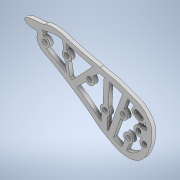
# Autodesk Inventor part: Component26
Saved by Autodesk Inventor 2022 (Build 260153000, 153)
## iProperties
Created: 2022-01-29
Part Number: Component26
Material: Generic
Document SubType Name: Modeling
Designer: Administrator
Density: 1 g/cm^3
Appearance: Default
Title: Component26
Author: Administrator
Autodesk Inventor part; units mm, degrees
ref_plane "YZ Plane" through (0, 0, 0) normal (1, 0, 0) x (0, 1, 0)
ref_plane "XZ Plane" through (0, 0, 0) normal (0, 1, 0) x (-1, 0, 0)
ref_plane "XY Plane" through (0, 0, 0) normal (0, 0, 1) x (1, 0, 0)
sketch "Sketch4" plane through (0, 0, 0) normal (0, 0, 1) x (1, 0, 0)
  circle A0 centre (-123.2659, 62.3625) radius 3.25
  circle A1 centre (-93.6225, 61.5254) radius 3.25
  circle A2 centre (-63.1067, 48.9642) radius 3.25
  circle A3 centre (-41.8815, 23.3302) radius 6.6019
  circle A4 centre (-41.8815, 23.3302) radius 3.25
  circle A5 centre (-63.1067, 48.9642) radius 6.8839
  circle A6 centre (-93.6225, 61.5254) radius 6.35
  circle A7 centre (-123.2659, 62.3625) radius 6.35
  circle A8 centre (-17.9295, 30.4928) radius 3.25
  circle A9 centre (-17.9295, 30.4928) radius 6.3607
  arc A10 (-9.0364, 0.4347) -> (-15.1641, 2.1132) centre (-10.6476, 6.5768) ccw
  circle A11 centre (-10.6476, 6.5768) radius 3.25
  circle A12 centre (-10.6476, 6.5768) radius 6.35
  circle A13 centre (3.2167, 21.804) radius 3.25
  circle A14 centre (3.2167, 21.804) radius 6.3938
  circle A15 centre (11.1828, 10.2103) radius 3.25
  circle A16 centre (11.1828, 10.2103) radius 6.35
  line L0 (0.487, 42.0553) -> (6.4199, 38.5891) construction
  line L1 (0.487, 42.0553) -> (6.4199, 38.5891) construction
  line L2 (-99.3839, 77.1398) -> (-97.7962, 66.3111)
  line L3 (-99.3839, 77.1398) -> (-97.7962, 66.3111)
  line L4 (-94.4581, 75.1449) -> (-93.4037, 67.8716)
  line L5 (-94.4581, 75.1449) -> (-93.4037, 67.8716)
  line L6 (-89.1475, 38.513) -> (-91.9311, 53.8666)
  line L7 (-92.1978, 55.3373) -> (-89.1475, 38.513)
  line L8 (-44.7292, 29.2864) -> (-43.2829, 61.21)
  line L9 (-43.2829, 61.21) -> (-44.7292, 29.2864)
  line L10 (-37.6136, 1.1054) -> (-18.29, 54.3043)
  line L11 (-16.6773, 36.7291) -> (-11.0974, 52.1068)
  line L12 (-11.0974, 52.1068) -> (-16.6773, 36.7291)
  line L13 (-30.4763, -2.5717) -> (-20.5684, 24.7053)
  line L14 (-20.5684, 24.7053) -> (-30.4763, -2.5717)
  line L15 (-15.1641, 2.1132) -> (-18.9648, -7.672)
  line L16 (-15.1641, 2.1132) -> (-18.9648, -7.672)
  line L17 (-12.6206, -8.9306) -> (-9.0364, 0.4347)
  line L18 (-9.0364, 0.4347) -> (-12.6206, -8.9306)
  spline S0 degree 1 poles (-89.1475, 38.513) (-86.314, 36.5681) knots 0 0 1 1
  spline S1 degree 3 poles (-94.4581, 75.1449) (-89.0039, 73.5308) (-61.0651, 66.1302) (-58.348, 66.0513) knots 0 0 0 0 1 1 1 1
  spline S2 degree 2 poles (-124.9306, 68.4904) (-124.7941, 71.5671) (-126.6326, 74.9703) knots 0 0 0 1 1 1
  spline S3 degree 4 poles (-126.6326, 74.9703) (-124.6811, 75.0735) (-123.6465, 74.6991) (-116.9052, 77.5165) (-111.8408, 77.8952) (-106.9644, 78.3944) (-102.5411, 77.5396) (-100.8183, 77.334) (-99.3839, 77.1398) knots 0 0 0 0 0 0.325065 0.476889 0.636712 0.785428 1 1 1 1 1
  line L19 (-102.3701, 77.544) -> (-96.3977, 76.7356) construction
  arc A17 (-96.9973, 76.8008) -> (-101.7747, 77.4475) centre (-124.0221, -104.8878) ccw construction
  spline S4 degree 4 poles (-79.9023, 31.8379) (-68.677, 24.1558) (-65.7048, 21.8411) (-54.4696, 13.1783) (-47.2097, 8.1156) knots 0 0 0 0 0 1 1 1 1 1
  line L20 (-36.0787, 59.4886) -> (-37.5047, 28.2728)
  spline S5 degree 1 poles (-50.2018, 62.6533) (-43.2829, 61.21) knots 0 0 1 1
  line L21 (-58.8336, 54.3613) -> (-50.2018, 62.6533)
  spline S6 degree 4 poles (-48.4944, 70.2012) (-36.0141, 65.7072) (-30.7305, 68.7389) (-7.2655, 57.0667) (9.3089, 53.4776) (21.1008, 36.626) (20.9729, 33.2176) (20.9498, 16.3118) (19.6092, 12.859) (15.3586, 0.2622) (11.6074, -5.1677) (4.6087, -13.37) (-6.6845, -16.5209) (-13.4963, -16.6569) (-26.6726, -14.6721) (-37.9818, -6.8681) (-48.5195, -2.2945) (-56.5284, 5.7043) (-68.3866, 14.707) (-76.2345, 20.2103) (-90.2288, 29.4992) (-101.4213, 37.2305) (-118.0489, 46.4365) (-128.5275, 50.5525) (-133.6617, 58.8987) (-134.3025, 63.1982) (-132.382, 69.7186) (-133.4886, 70.4797) (-138.3156, 70.5557) (-142.305, 70.8214) (-145.7075, 71.2674) (-149.1406, 73.4071) (-150.5992, 74.9837) (-150.3106, 77.5083) (-148.4094, 78.2404) (-147.041, 79.3341) (-144.1806, 80.1808) (-141.6683, 80.7774) (-137.5469, 81.2031) (-134.4054, 81.6387) (-131.7323, 81.4914) (-129.0357, 81.5666) (-125.9455, 82.1526) (-124.1195, 82.6025) (-123.0686, 83.1991) knots 0 0 0 0 0 0.084441 0.118474 0.150262 0.180443 0.207707 0.233569 0.259946 0.285424 0.312388 0.338232 0.365444 0.393991 0.422871 0.453116 0.483798 0.513365 0.543967 0.576006 0.609621 0.643558 0.675095 0.702806 0.725607 0.743321 0.759311 0.775075 0.790518 0.807822 0.823963 0.838322 0.851216 0.862814 0.874845 0.887711 0.90222 0.917813 0.933276 0.94829 0.962767 0.97721 1 1 1 1 1
  line L22 (-67.7671, 43.8978) -> (-79.9023, 31.8379)
  line L23 (-96.2693, 55.7533) -> (-93.9578, 41.2636)
  spline S7 degree 4 poles (-121.1299, 56.3826) (-112.9596, 50.6322) (-106.8288, 48.999) (-98.1791, 43.4387) (-93.9578, 41.2636) knots 0 0 0 0 0 1 1 1 1 1
  spline S8 degree 3 poles (-36.0787, 59.4886) (-32.0611, 58.7648) (-23.4035, 55.5205) (-18.29, 54.3043) knots 0 0 0 0 1 1 1 1
  line L24 (-38.7053, 2.6027) -> (-38.0024, 17.9881)
  spline S9 degree 4 poles (-123.0686, 83.1991) (-121.5996, 84.0331) (-117.1799, 84.5502) (-116.7574, 85.3349) (-102.0621, 84.8359) (-94.4012, 81.5385) (-82.7685, 78.513) (-69.5272, 74.408) (-54.1219, 71.5671) (-48.4944, 70.2012) knots 0 0 0 0 0 0.116866 0.21775 0.322652 0.463158 0.611266 1 1 1 1 1
  line L25 (-122.3958, 83.8471) -> (-111.8454, 85.6152) construction
  arc A18 (-112.8875, 85.1999) -> (-121.2753, 83.7942) centre (-110.8052, 47.0461) ccw construction
  line L26 (13.5332, 27.0791) -> (5.6, 27.7371)
  spline S10 degree 3 poles (13.5332, 27.0791) (17.0401, 28.2955) (11.4801, 33.321) (12.1713, 35.8976) knots 0 0 0 0 1 1 1 1
  spline S11 degree 4 poles (-12.6206, -8.9306) (-11.0988, -9.1567) (-7.9065, -8.9799) (-0.7866, -6.5594) (4.7218, -1.6082) (7.094, 3.0589) (8.3854, 4.5096) knots 0 0 0 0 0 0.301338 0.510276 1 1 1 1 1
  line L27 (-47.2097, 8.1156) -> (-46.7199, 18.8384)
  spline S12 degree 1 poles (-38.7053, 2.6027) (-37.6136, 1.1054) knots 0 0 1 1
  spline S13 degree 4 poles (-30.4763, -2.5717) (-29.8635, -4.0953) (-23.7582, -5.4905) (-22.3176, -7.1502) (-18.9648, -7.672) knots 0 0 0 0 0 1 1 1 1 1
  line L28 (0.487, 42.0553) -> (6.4199, 38.5891) construction
  line L29 (-2.7162, 36.5725) -> (3.2167, 33.1063)
  line L30 (9.6232, 44.072) -> (3.6902, 47.5382)
  arc A19 (3.6902, 47.5382) -> (-2.7162, 36.5725) centre (0.487, 42.0553) ccw
  arc A20 (3.2167, 33.1063) -> (9.6232, 44.072) centre (6.4199, 38.5891) ccw
  spline S14 degree 4 poles (-11.0974, 52.1068) (-10.8972, 52.6451) (-5.9101, 48.9599) (-3.1879, 49.4055) (-2.1589, 47.8278) knots 0 0 0 0 0 1 1 1 1 1
  line L31 (0.487, 42.0553) -> (6.4199, 38.5891) construction
  line L32 (2.1265, 44.8615) -> (8.0594, 41.3953)
  line L33 (4.7805, 35.7829) -> (-1.1524, 39.2491)
  arc A21 (2.1265, 44.8615) -> (-1.1524, 39.2491) centre (0.487, 42.0553) ccw
  arc A22 (4.7805, 35.7829) -> (8.0594, 41.3953) centre (6.4199, 38.5891) ccw
  line L34 (-86.314, 36.5681) -> (-58.348, 66.0513)
  line L35 (3.2167, 15.4102) -> (7.5381, 15.4102)
  line L36 (-15.1406, -8.5562) -> (-10.1007, -9.3049) construction
  arc A23 (-14.5441, -8.404) -> (-10.6272, -8.9859) centre (-11.3942, -0.6747) ccw construction
  point P0 (0, 0)
  point P1 (3.4535, 40.3222)
  point P2 (3.4535, 40.3222)
  point P3 (-83.197, 72.0665)
  point P4 (-63.3289, 67.0346)
  point P5 (-125.2394, 71.4578)
  point P6 (-124.5026, 75.0553)
  point P7 (-121.6588, 75.6416)
  point P8 (-116.0905, 77.2602)
  point P9 (-111.6668, 77.9259)
  point P10 (-107.1522, 78.0845)
  point P11 (-102.5828, 77.5823)
  point P12 (-63.3283, 19.9895)
  point P13 (-67.6095, 14.019)
  point P14 (-70.2118, 25.0604)
  point P15 (-55.2549, 13.9519)
  point P16 (-33.4871, 66.5925)
  point P17 (-20.6666, 63.2711)
  point P18 (-3.0393, 56.784)
  point P19 (10.3795, 49.6099)
  point P20 (19.697, 37.3317)
  point P21 (20.9543, 30.7069)
  point P22 (20.585, 17.8397)
  point P23 (19.1683, 11.5104)
  point P24 (15.3531, 1.4868)
  point P25 (11.1804, -5.3901)
  point P26 (3.8615, -12.2784)
  point P27 (-5.9583, -15.9225)
  point P28 (-13.5398, -16.304)
  point P29 (-25.3402, -13.8592)
  point P30 (-38.1309, -7.3256)
  point P31 (-48.0759, -1.557)
  point P32 (-57.007, 5.6696)
  point P33 (-76.3522, 20.2082)
  point P34 (-88.7766, 28.5824)
  point P35 (-102.5781, 37.5478)
  point P36 (-119.6247, 46.8159)
  point P37 (-129.4025, 53.2681)
  point P38 (-133.3877, 59.7383)
  point P39 (-133.6123, 64.9346)
  point P40 (-132.9983, 69.4096)
  point P41 (-133.7787, 70.2207)
  point P42 (-137.5911, 70.5697)
  point P43 (-142.3147, 70.8802)
  point P44 (-146.1131, 71.7837)
  point P45 (-149.2626, 73.7357)
  point P46 (-150.3083, 75.4489)
  point P47 (-149.9428, 77.2311)
  point P48 (-148.6086, 78.2495)
  point P49 (-147.089, 79.1182)
  point P50 (-144.6312, 80.0215)
  point P51 (-141.6917, 80.6837)
  point P52 (-137.4889, 81.2333)
  point P53 (-134.1664, 81.5354)
  point P54 (-131.7413, 81.5337)
  point P55 (-129.4102, 81.6346)
  point P56 (-126.1766, 82.1503)
  point P57 (-98.1366, 43.5746)
  point P58 (-104.7791, 47.205)
  point P59 (-112.3268, 51.1181)
  point P60 (-24.4257, 56.0733)
  point P61 (-31.6333, 58.3402)
  point P62 (-61.0372, 72.9432)
  point P63 (-86.731, 79.4913)
  point P64 (-106.3338, 84.6959)
  point P65 (-117.1206, 84.7312)
  point P66 (-94.4887, 81.835)
  point P67 (-76.4524, 76.6451)
  point P68 (14.6933, 28.7644)
  point P69 (13.081, 32.5705)
  point P70 (-25.3388, -5.3867)
  point P71 (-21.946, -6.8042)
  point P72 (6.3564, 1.6685)
  point P73 (2.6486, -2.8719)
  point P74 (-2.5579, -6.6485)
  point P75 (-12.666, -8.9237)
  point P76 (-29.0617, -3.7189)
  point P77 (3.4535, 40.3222)
  point P78 (-10.7812, 52.1086)
  point P79 (-7.5998, 50.59)
  point P80 (-3.665, 48.9029)
  point P81 (3.4535, 40.3222)
  point P82 (-44.45, 61.9125)
  point P83 (-92.0343, 55.4942)
  point P84 (12.1713, 35.8976)
  point P85 (8.2264, 4.5905)
  point P86 (-12.666, -8.7985)
  point P87 (-18.9648, -7.672)
  point P88 (-31.4568, -2.4563)
  point P89 (-120.9781, 56.439)
  point P90 (-18.8701, 54.5151)
  point P91 (-38.1296, 1.4925)
  dimension "d2" = 6.5
  dimension "d3" = 25
  dimension "d4" = 25
  dimension "d6" = 33
  constraints: 82 end point, 33 point on circle, 24 centre point, 10 collinear, 10 midpoint, 9 equal radius, 9 tangent, 7 coincident, 2 parallel, 1 concentric, 1 horizontal, 117 other
  measures "d2" diameter of A2
  measures "d3" distance of A11.centre A9.centre
  measures "d4" distance of A3.centre A9.centre
  measures "d6" distance of A1.centre A5.centre
extrude "Extrusion1" add sketch "Sketch4" along normal blind 5 contours A3 | A5 | A6 | A7 | A9 | A19 L30 A20 L29 | A10 A12 | A16 | A14 | S6 S9
equation "\"d2\" = R"
equation "\"d0\" = thickness"
equation "\"R\" = 6.5"
equation "\"thickness\" = 5"
equation "\"width\" = 6.5"
equation "\"R1\" = 9"
body "Solid2"
